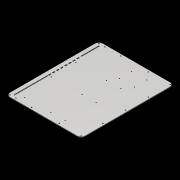
# Autodesk Inventor part: right_panel
Saved by Autodesk Inventor 2018.2 (Build 222227000, 227)
## iProperties
Created: 2019-10-14
Part Number: right_panel
Material: アルミニウム 6061
Document SubType Name: Modeling
Designer: gisen
Density: 2.7 g/cm^3
Appearance: アルミニウム - フラット
Author: gisen
Autodesk Inventor part; units mm, degrees
ref_plane "YZ Plane" through (0, 0, 0) normal (1, 0, 0) x (0, 1, 0)
ref_plane "XZ Plane" through (0, 0, 0) normal (0, 1, 0) x (-1, 0, 0)
ref_plane "XY Plane" through (0, 0, 0) normal (0, 0, 1) x (1, 0, 0)
sketch "スケッチ1" plane through (0, 0, 0) normal (0, 0, 1) x (1, 0, 0)
  line L0 (-170, -235) -> (170, -235)
  line L1 (190, -215) -> (190, 215)
  line L2 (170, 235) -> (-170, 235)
  line L3 (-190, 215) -> (-190, -215)
  line L4 (-190, -235) -> (190, 235) construction
  line L5 (190, -235) -> (-190, 235) construction
  circle A0 centre (-180, 225) radius 2.25
  circle A1 centre (180, 225) radius 2.25
  circle A2 centre (-180, -225) radius 2.25
  circle A3 centre (180, -225) radius 2.25
  arc A4 (-170, 235) -> (-190, 215) centre (-170, 215) ccw
  arc A5 (190, 215) -> (170, 235) centre (170, 215) ccw
  arc A6 (170, -235) -> (190, -215) centre (170, -215) ccw
  arc A7 (-190, -215) -> (-170, -235) centre (-170, -215) ccw
  point P0 (0, 0)
  dimension "d0" = 380
  dimension "d1" = 470
  dimension "d2" = 4.5
  dimension "d3" = 10
  dimension "d4" = 10
  dimension "d5" = 10
  dimension "d6" = 10
  dimension "d7" = 10
  dimension "d8" = 10
  dimension "d9" = 10
  dimension "d10" = 10
  dimension "d11" = 20
  constraints: 12 end point, 8 centre point, 8 point on circle, 8 point on line, 8 tangent, 6 equal radius, 2 midpoint, 2 parallel, 1 horizontal, 1 perpendicular
  measures "d0" distance of L5.end L4.end
  measures "d1" distance of L4.end L5.start
  measures "d2" diameter of A0
  measures "d3" distance from line of A0.centre L2
  measures "d4" distance from line of L3 A0.centre
  measures "d5" distance from line of A1.centre L2
  measures "d6" distance from line of L1 A1.centre
  measures "d7" distance from line of L1 A3.centre
  measures "d8" distance from line of L0 A3.centre
  measures "d9" distance from line of L0 A2.centre
  measures "d10" distance from line of L3 A2.centre
  measures "d11" radius of A4
extrude "押し出し1" add sketch "スケッチ1" along normal blind 3
sketch "スケッチ2" plane through (0, 0, 3) normal (0, 0, 1) x (1, 0, 0)
  circle A0 centre (73.0923, -199.0135) radius 2.25 construction
  circle A1 centre (-131.3777, -199.0135) radius 2.25 construction
  circle A2 centre (73.0923, -41.5335) radius 2.25 construction
  circle A3 centre (73.0923, 82.9265) radius 2.25 construction
  circle A4 centre (0.7023, -199.0135) radius 2.25 construction
  circle A5 centre (0.7023, -41.5335) radius 2.25 construction
  circle A6 centre (0.7023, 82.9265) radius 2.25 construction
  circle A7 centre (-154.2377, -41.5335) radius 2.25 construction
  circle A8 centre (-154.2377, 82.9265) radius 2.25 construction
  circle A9 centre (73.0923, 82.9265) radius 1.6
  circle A10 centre (0.7023, 82.9265) radius 1.6
  circle A11 centre (-154.2377, 82.9265) radius 1.6
  circle A12 centre (-154.2377, -41.5335) radius 1.6
  circle A13 centre (-131.3777, -199.0135) radius 1.6
  circle A14 centre (0.7023, -199.0135) radius 1.6
  circle A15 centre (73.0923, -199.0135) radius 1.6
  circle A16 centre (73.0923, -41.5335) radius 1.6
  circle A17 centre (0.7023, -41.5335) radius 1.6
  point P0 (0, 0)
  dimension "d14" = 3.2
  constraints: 9 centre point, 9 coincident, 8 equal radius
  measures "d14" diameter of A9
extrude "押し出し2" cut sketch "スケッチ2" against normal blind 3
sketch "スケッチ4" plane through (0, 0, 3) normal (0, 0, 1) x (1, 0, 0)
  line L0 (-170, -215) -> (-170, -46.0635) projected
  line L1 (-170, -215) -> (-167, -215) projected
  line L2 (-167, -46.0635) -> (-167, -215) projected
  line L3 (-170, -46.0635) -> (-167, -46.0635) projected
  line L4 (-170, -40.8932) -> (-170, -30.6062) projected
  line L5 (-170, -40.8932) -> (-167, -40.8932) projected
  line L6 (-167, -30.6062) -> (-167, -40.8932) projected
  line L7 (-170, -30.6062) -> (-167, -30.6062) projected
  line L8 (-170, -20.5478) -> (-170, -10.2608) projected
  line L9 (-170, -20.5478) -> (-167, -20.5478) projected
  line L10 (-167, -10.2608) -> (-167, -20.5478) projected
  line L11 (-170, -10.2608) -> (-167, -10.2608) projected
  line L12 (-170, 0.1068) -> (-170, 10.3938) projected
  line L13 (-170, 0.1068) -> (-167, 0.1068) projected
  line L14 (-167, 10.3938) -> (-167, 0.1068) projected
  line L15 (-170, 10.3938) -> (-167, 10.3938) projected
  line L16 (-170, 20.4522) -> (-170, 30.7392) projected
  line L17 (-170, 20.4522) -> (-167, 20.4522) projected
  line L18 (-167, 30.7392) -> (-167, 20.4522) projected
  line L19 (-170, 30.7392) -> (-167, 30.7392) projected
  line L20 (-170, 41.1068) -> (-170, 51.3938) projected
  line L21 (-170, 41.1068) -> (-167, 41.1068) projected
  line L22 (-167, 51.3938) -> (-167, 41.1068) projected
  line L23 (-170, 51.3938) -> (-167, 51.3938) projected
  line L24 (-170, 61.4522) -> (-170, 71.7392) projected
  line L25 (-170, 61.4522) -> (-167, 61.4522) projected
  line L26 (-167, 71.7392) -> (-167, 61.4522) projected
  line L27 (-170, 71.7392) -> (-167, 71.7392) projected
  line L28 (-170, 82.1068) -> (-170, 92.3938) projected
  line L29 (-170, 82.1068) -> (-167, 82.1068) projected
  line L30 (-167, 92.3938) -> (-167, 82.1068) projected
  line L31 (-170, 92.3938) -> (-167, 92.3938) projected
  line L32 (-170, 102.4522) -> (-170, 112.7392) projected
  line L33 (-170, 102.4522) -> (-167, 102.4522) projected
  line L34 (-167, 112.7392) -> (-167, 102.4522) projected
  line L35 (-170, 112.7392) -> (-167, 112.7392) projected
  line L36 (-170, 215) -> (-170, 124.6) projected
  line L37 (-170, 124.6) -> (-167, 124.6) projected
  line L38 (-167, 215) -> (-167, 124.6) projected
  line L39 (-170, 215) -> (-167, 215) projected
  line L40 (-167, 112.7392) -> (-166, 112.7392)
  line L41 (-166, 112.7392) -> (-166, 102.4522)
  line L42 (-166, 102.4522) -> (-167, 102.4522)
  line L43 (-167, 92.3938) -> (-166, 92.3938)
  line L44 (-166, 92.3938) -> (-166, 82.1068)
  line L45 (-166, 82.1068) -> (-167, 82.1068)
  line L46 (-167, 71.7392) -> (-166, 71.7392)
  line L47 (-166, 71.7392) -> (-166, 61.4522)
  line L48 (-166, 61.4522) -> (-167, 61.4522)
  line L49 (-167, 51.3938) -> (-166, 51.3938)
  line L50 (-166, 51.3938) -> (-166, 41.1068)
  line L51 (-166, 41.1068) -> (-167, 41.1068)
  line L52 (-167, 30.7392) -> (-166, 30.7392)
  line L53 (-166, 30.7392) -> (-166, 20.4522)
  line L54 (-166, 20.4522) -> (-167, 20.4522)
  line L55 (-167, 10.3938) -> (-166, 10.3938)
  line L56 (-166, 10.3938) -> (-166, 0.1068)
  line L57 (-166, 0.1068) -> (-167, 0.1068)
  line L58 (-167, -10.2608) -> (-166, -10.2608)
  line L59 (-166, -10.2608) -> (-166, -20.5478)
  line L60 (-166, -20.5478) -> (-167, -20.5478)
  line L61 (-167, -30.6062) -> (-166, -30.6062)
  line L62 (-166, -30.6062) -> (-166, -40.8932)
  line L63 (-166, -40.8932) -> (-167, -40.8932)
  point P0 (0, 0)
  dimension "d17" = 1
  constraints: 48 end point, 15 perpendicular, 8 horizontal, 7 parallel, 1 collinear
  measures "d17" distance of L34.start L40.end
extrude "押し出し3" cut sketch "スケッチ4" against normal blind 3
sketch "スケッチ5" plane through (0, 0, 3) normal (0, 0, 1) x (1, 0, 0)
  circle A0 centre (-180, 225) radius 2.25 construction
  circle A1 centre (-180, -225) radius 2.25 construction
  circle A2 centre (-150, -225) radius 2.25
  line L0 (-170, -235) -> (170, -235) projected
  circle A3 centre (-150, 225) radius 2.25
  line L1 (170, 235) -> (-170, 235) projected
  point P0 (0, 0)
  dimension "d20" = 30
  dimension "d21" = 10
  dimension "d22" = 30
  dimension "d23" = 10
  constraints: 2 centre point, 2 equal radius
  measures "d20" distance of A1.centre A2.centre
  measures "d21" distance from line of L0 A2.centre
  measures "d22" distance of A0.centre A3.centre
  measures "d23" distance from line of L1 A3.centre
extrude "押し出し4" cut sketch "スケッチ5" against normal blind 3
sketch "スケッチ6" plane through (0, 0, 3) normal (0, 0, 1) x (1, 0, 0)
  circle A0 centre (-150, -225) radius 2.25 construction
  circle A1 centre (-150, 225) radius 2.25 construction
  line L0 (-167, 124.6) -> (-170, 124.6) construction
  line L1 (-170, 124.6) -> (-170, 215) construction
  line L2 (-170, 215) -> (-167, 215) construction
  line L3 (-167, 215) -> (-167, 124.6) construction
  line L4 (-166, 92.3938) -> (-166, 82.1068) construction
  line L5 (-166, 82.1068) -> (-170, 82.1068) construction
  line L6 (-170, 82.1068) -> (-170, 92.3938) construction
  line L7 (-170, 92.3938) -> (-166, 92.3938) construction
  line L8 (-166, 51.3938) -> (-166, 41.1068) construction
  line L9 (-166, 41.1068) -> (-170, 41.1068) construction
  line L10 (-170, 41.1068) -> (-170, 51.3938) construction
  line L11 (-170, 51.3938) -> (-166, 51.3938) construction
  line L12 (-166, 10.3938) -> (-166, 0.1068) construction
  line L13 (-166, 0.1068) -> (-170, 0.1068) construction
  line L14 (-170, 0.1068) -> (-170, 10.3938) construction
  line L15 (-170, 10.3938) -> (-166, 10.3938) construction
  line L16 (-166, -30.6062) -> (-166, -40.8932) construction
  line L17 (-166, -40.8932) -> (-170, -40.8932) construction
  line L18 (-170, -40.8932) -> (-170, -30.6062) construction
  line L19 (-170, -30.6062) -> (-166, -30.6062) construction
  line L20 (-166, -10.2608) -> (-166, -20.5478) construction
  line L21 (-166, -20.5478) -> (-170, -20.5478) construction
  line L22 (-170, -20.5478) -> (-170, -10.2608) construction
  line L23 (-170, -10.2608) -> (-166, -10.2608) construction
  line L24 (-166, 30.7392) -> (-166, 20.4522) construction
  line L25 (-166, 20.4522) -> (-170, 20.4522) construction
  line L26 (-170, 20.4522) -> (-170, 30.7392) construction
  line L27 (-170, 30.7392) -> (-166, 30.7392) construction
  line L28 (-166, 71.7392) -> (-166, 61.4522) construction
  line L29 (-166, 61.4522) -> (-170, 61.4522) construction
  line L30 (-170, 61.4522) -> (-170, 71.7392) construction
  line L31 (-170, 71.7392) -> (-166, 71.7392) construction
  line L32 (-166, 112.7392) -> (-166, 102.4522) construction
  line L33 (-166, 102.4522) -> (-170, 102.4522) construction
  line L34 (-170, 102.4522) -> (-170, 112.7392) construction
  line L35 (-170, 112.7392) -> (-166, 112.7392) construction
  line L36 (-167, -215) -> (-170, -215) construction
  line L37 (-170, -215) -> (-170, -46.0635) construction
  line L38 (-170, -46.0635) -> (-167, -46.0635) construction
  line L39 (-167, -46.0635) -> (-167, -215) construction
  circle A2 centre (73.0923, -41.5335) radius 1.6 construction
  circle A3 centre (0.7023, -199.0135) radius 1.6 construction
  circle A4 centre (-154.2377, -41.5335) radius 1.6 construction
  circle A5 centre (0.7023, 82.9265) radius 1.6 construction
  circle A6 centre (73.0923, 82.9265) radius 1.6 construction
  circle A7 centre (-154.2377, 82.9265) radius 1.6 construction
  circle A8 centre (-131.3777, -199.0135) radius 1.6 construction
  circle A9 centre (73.0923, -199.0135) radius 1.6 construction
  circle A10 centre (0.7023, -41.5335) radius 1.6 construction
  circle A11 centre (180, -225) radius 2.25 construction
  circle A12 centre (-180, -225) radius 2.25 construction
  circle A13 centre (180, 225) radius 2.25 construction
  circle A14 centre (-180, 225) radius 2.25 construction
  line L40 (170, 235) -> (-170, 235) construction
  arc A15 (-170, 235) -> (-190, 215) centre (-170, 215) ccw construction
  line L41 (-190, 215) -> (-190, -215) construction
  arc A16 (-190, -215) -> (-170, -235) centre (-170, -215) ccw construction
  line L42 (-170, -235) -> (170, -235) construction
  arc A17 (170, -235) -> (190, -215) centre (170, -215) ccw construction
  line L43 (190, -215) -> (190, 215) construction
  arc A18 (190, 215) -> (170, 235) centre (170, 215) ccw construction
  line L44 (-166.75, 124.35) -> (-170.25, 124.35)
  line L45 (-170.25, 124.35) -> (-170.25, 215.25)
  line L46 (-170.25, 215.25) -> (-166.75, 215.25)
  line L47 (-166.75, 215.25) -> (-166.75, 124.35)
  line L48 (-165.75, 112.9892) -> (-165.75, 102.2022)
  line L49 (-165.75, 102.2022) -> (-170.25, 102.2022)
  line L50 (-170.25, 102.2022) -> (-170.25, 112.9892)
  line L51 (-170.25, 112.9892) -> (-165.75, 112.9892)
  line L52 (-165.75, 92.6438) -> (-165.75, 81.8568)
  line L53 (-165.75, 81.8568) -> (-170.25, 81.8568)
  line L54 (-170.25, 81.8568) -> (-170.25, 92.6438)
  line L55 (-170.25, 92.6438) -> (-165.75, 92.6438)
  line L56 (-165.75, 71.9892) -> (-165.75, 61.2022)
  line L57 (-165.75, 61.2022) -> (-170.25, 61.2022)
  line L58 (-170.25, 61.2022) -> (-170.25, 71.9892)
  line L59 (-170.25, 71.9892) -> (-165.75, 71.9892)
  line L60 (-165.75, 51.6438) -> (-165.75, 40.8568)
  line L61 (-165.75, 40.8568) -> (-170.25, 40.8568)
  line L62 (-170.25, 40.8568) -> (-170.25, 51.6438)
  line L63 (-170.25, 51.6438) -> (-165.75, 51.6438)
  line L64 (-165.75, 30.9892) -> (-165.75, 20.2022)
  line L65 (-165.75, 20.2022) -> (-170.25, 20.2022)
  line L66 (-170.25, 20.2022) -> (-170.25, 30.9892)
  line L67 (-170.25, 30.9892) -> (-165.75, 30.9892)
  line L68 (-165.75, 10.6438) -> (-165.75, -0.1432)
  line L69 (-165.75, -0.1432) -> (-170.25, -0.1432)
  line L70 (-170.25, -0.1432) -> (-170.25, 10.6438)
  line L71 (-170.25, 10.6438) -> (-165.75, 10.6438)
  line L72 (-165.75, -10.0108) -> (-165.75, -20.7978)
  line L73 (-165.75, -20.7978) -> (-170.25, -20.7978)
  line L74 (-170.25, -20.7978) -> (-170.25, -10.0108)
  line L75 (-170.25, -10.0108) -> (-165.75, -10.0108)
  line L76 (-165.75, -30.3562) -> (-165.75, -41.1432)
  line L77 (-165.75, -41.1432) -> (-170.25, -41.1432)
  line L78 (-170.25, -41.1432) -> (-170.25, -30.3562)
  line L79 (-170.25, -30.3562) -> (-165.75, -30.3562)
  line L80 (-166.75, -45.8135) -> (-170.25, -45.8135)
  line L81 (-170.25, -45.8135) -> (-170.25, -215.25)
  line L82 (-170.25, -215.25) -> (-166.75, -215.25)
  line L83 (-166.75, -215.25) -> (-166.75, -45.8135)
  point P0 (0, 0)
  dimension "d26" = 0.25
  dimension "d27" = 0.25
  dimension "d28" = 0.25
  dimension "d29" = 0.25
  dimension "d30" = 0.25
  dimension "d31" = 0.25
  dimension "d32" = 0.25
  dimension "d33" = 0.25
  dimension "d34" = 0.25
  dimension "d35" = 0.25
  constraints: 80 end point, 30 other
  measures "d26" distance between parallel lines of L3 L47
  measures "d27" distance between parallel lines of L35 L51
  measures "d28" distance between parallel lines of L7 L55
  measures "d29" distance between parallel lines of L31 L59
  measures "d30" distance between parallel lines of L11 L63
  measures "d31" distance between parallel lines of L27 L67
  measures "d32" distance between parallel lines of L15 L71
  measures "d33" distance between parallel lines of L23 L75
  measures "d34" distance between parallel lines of L19 L79
  measures "d35" distance between parallel lines of L38 L80
extrude "押し出し5" cut sketch "スケッチ6" against normal through all
sketch "スケッチ7" plane through (0, 0, 3) normal (0, 0, 1) x (1, 0, 0)
  line L0 (190, 215) -> (190, -215) projected
  circle A0 centre (-70, -225) radius 2.25 projected
  circle A1 centre (180, 0) radius 2.25 projected
  circle A2 centre (70, -225) radius 2.25 projected
  circle A3 centre (180, 115) radius 2.25 projected
  circle A4 centre (-70, 225) radius 2.25 projected
  circle A5 centre (-180, -115) radius 2.25 projected
  circle A6 centre (-180, 0) radius 2.25 projected
  circle A7 centre (70, 225) radius 2.25 projected
  circle A8 centre (180, -115) radius 2.25 projected
  line L1 (-170.2, 124.4) -> (-166.8, 124.4) projected
  line L2 (-166.8, 124.4) -> (-166.8, 215.2) projected
  line L3 (-166.8, 215.2) -> (-170.2, 215.2) projected
  line L4 (-170.2, 215.2) -> (-170.2, 124.4) projected
  circle A9 centre (-180, 115) radius 2.25 projected
  circle A10 centre (180, 225) radius 2.25 projected
  circle A11 centre (-180, 225) radius 2.25 projected
  circle A12 centre (180, -225) radius 2.25 projected
  circle A13 centre (-180, -225) radius 2.25 projected
  line L5 (170, -235) -> (-170, -235) projected
  arc A14 (-190, -215) -> (-170, -235) centre (-170, -215) ccw projected
  line L6 (-190, -215) -> (-190, 215) projected
  arc A15 (-170, 235) -> (-190, 215) centre (-170, 215) ccw projected
  line L7 (-170, 235) -> (170, 235) projected
  arc A16 (190, 215) -> (170, 235) centre (170, 215) ccw projected
  line L8 (190, 215) -> (190, -215) projected
  arc A17 (170, -235) -> (190, -215) centre (170, -215) ccw projected
  point P0 (0, 0)
extrude "押し出し6" cut sketch "スケッチ7" against normal up to surface (3 mm away) contours A0 | A1 | A2 | A3 | A4 | A7 | A8
sketch "スケッチ8" plane through (0, 0, 0) normal (0, 0, -1) x (-1, 0, 0)
  line L0 (-14.775, 120.075) -> (-115.225, 120.075) construction
  line L1 (-115.225, 120.075) -> (-115.225, 189.925) construction
  line L2 (-115.225, 189.925) -> (-14.775, 189.925) construction
  line L3 (-14.775, 189.925) -> (-14.775, 120.075) construction
  line L4 (-14.775, 120.075) -> (-115.225, 189.925) construction
  line L5 (-115.225, 120.075) -> (-14.775, 189.925) construction
  line L6 (170, 235) -> (-170, 235) construction
  line L7 (-190, 215) -> (-190, -215) construction
  line L8 (-24.625, 185.86) -> (-101.225, 185.86) construction
  line L9 (-101.225, 185.86) -> (-101.225, 124.14) construction
  line L10 (-101.225, 124.14) -> (-24.625, 124.14) construction
  line L11 (-24.625, 124.14) -> (-24.625, 185.86) construction
  line L12 (-24.625, 185.86) -> (-101.225, 124.14) construction
  line L13 (-101.225, 185.86) -> (-24.625, 124.14) construction
  line L14 (-62.925, 155) -> (-65, 155) construction
  circle A0 centre (-24.625, 124.14) radius 1.6
  circle A1 centre (-24.625, 185.86) radius 1.6
  circle A2 centre (-101.225, 185.86) radius 1.6
  circle A3 centre (-101.225, 124.14) radius 1.6
  point P0 (0, 0)
  dimension "d40" = 69.85
  dimension "d41" = 100.45
  dimension "d42" = 80
  dimension "d43" = 125
  dimension "d44" = 61.72
  dimension "d45" = 90.6
  dimension "d46" = 14
  dimension "d47" = 3.2
  dimension "d48" = 3.2
  dimension "d49" = 3.2
  dimension "d50" = 3.2
  constraints: 26 end point, 4 centre point, 4 coincident, 4 midpoint, 4 parallel, 3 horizontal, 2 perpendicular
  measures "d40" distance of L0.end L1.end
  measures "d41" distance of L0.start L0.end
  measures "d42" distance from line of L6 L14.end
  measures "d43" distance from line of L7 L14.end
  measures "d44" distance of L10.end L8.start
  measures "d45" distance between parallel lines of L1 L11
  measures "d46" distance between parallel lines of L1 L9
  measures "d47" diameter of A0
  measures "d48" diameter of A1
  measures "d49" diameter of A2
  measures "d50" diameter of A3
extrude "押し出し7" cut sketch "スケッチ8" against normal through all
equation "\"d5\" = d3"
equation "\"d6\" = d4"
equation "\"d7\" = d6"
equation "\"d8\" = d5"
equation "\"d9\" = d8"
equation "\"d10\" = d7"
